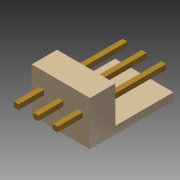
# Autodesk Inventor part: stiftleiste
Saved by Autodesk Inventor 2015 (Build 190159000, 159)
## iProperties
Created: 2015-03-02
Part Number: stiftleiste
Material: Generisch
Document SubType Name: Modeling
Designer: TowerSebi
Density: 1 g/cm^3
Appearance: Vorgabe
Author: TowerSebi
Autodesk Inventor part; units mm, degrees
ref_plane "YZ Plane" through (0, 0, 0) normal (1, 0, 0) x (0, 1, 0)
ref_plane "XZ Plane" through (0, 0, 0) normal (0, 1, 0) x (-1, 0, 0)
ref_plane "XY Plane" through (0, 0, 0) normal (0, 0, 1) x (1, 0, 0)
sketch "Skizze1" plane through (0, 0, 0) normal (0, 0, 1) x (1, 0, 0)
  line L0 (0, 0) -> (7.62, 0)
  line L1 (7.62, 0) -> (7.62, 3.3)
  line L2 (7.62, 3.3) -> (0, 3.3)
  line L3 (0, 3.3) -> (0, 0)
  dimension "d0" = 7.62
  dimension "d1" = 3.3
  constraints: 8 end point, 2 parallel, 1 horizontal, 1 perpendicular
  measures "d0" distance of L1.end L2.end
  measures "d1" distance of L2.end L0.start
extrude "Extrusion1" add sketch "Skizze1" along normal blind 5.8
sketch "Skizze2" plane through (0, 3.3, 0) normal (0, 1, 0) x (1, 0, 0)
  line L0 (7.62, 0) -> (7.62, -5.8) projected
  line L1 (0, 0) -> (7.62, 0)
  line L2 (7.62, 0) -> (7.62, -1)
  line L3 (7.62, -1) -> (0, -1)
  line L4 (0, -1) -> (0, 0)
  dimension "d4" = 1
  constraints: 8 end point, 2 parallel, 1 horizontal, 1 perpendicular, 1 point on line
  measures "d4" distance between parallel lines of L1 L3
extrude "Extrusion2" add sketch "Skizze2" along normal blind 7.6
sketch "Skizze3" plane through (0, 3.3, 5.8) normal (0, 1, 0) x (1, 0, 0)
  line L0 (7.62, 4.8) -> (0, 4.8) projected
  line L1 (0, 4.8) -> (0, 0) projected
  line L2 (7.62, 0) -> (0, 0) projected
  line L3 (7.62, 4.8) -> (7.62, 0) projected
  line L4 (0.95, 2.72) -> (1.59, 2.72)
  line L5 (1.59, 2.72) -> (1.59, 2.08)
  line L6 (1.59, 2.08) -> (0.95, 2.08)
  line L7 (0.95, 2.08) -> (0.95, 2.72)
  line L8 (3.49, 2.72) -> (4.13, 2.72)
  line L9 (4.13, 2.72) -> (4.13, 2.08)
  line L10 (4.13, 2.08) -> (3.49, 2.08)
  line L11 (3.49, 2.08) -> (3.49, 2.72)
  line L12 (6.03, 2.72) -> (6.67, 2.72)
  line L13 (6.67, 2.72) -> (6.67, 2.08)
  line L14 (6.67, 2.08) -> (6.03, 2.08)
  line L15 (6.03, 2.08) -> (6.03, 2.72)
  point P0 (0, 5.8)
  dimension "d7" = 0.64
  dimension "d8" = 0.64
  dimension "d9" = 0.64
  dimension "d10" = 0.64
  dimension "d11" = 0.64
  dimension "d12" = 0.64
  dimension "d13" = 7.62
  dimension "d15" = 1.9
  dimension "d16" = 1.9
  dimension "d17" = 0.95
  dimension "d18" = 0.95
  dimension "d19" = 4.8
  dimension "d20" = 2.08
  constraints: 24 end point, 6 parallel, 3 horizontal, 3 perpendicular
  measures "d7" distance of L14.end L12.start
  measures "d8" distance between parallel lines of L10 L8
  measures "d9" distance between parallel lines of L6 L4
  measures "d10" distance of L5.end L6.end
  measures "d11" distance of L13.end L14.end
  measures "d12" distance of L9.end L10.end
  measures "d13" distance between parallel lines of L3 L1
  measures "d15" distance between parallel lines of L11 L5
  measures "d16" distance between parallel lines of L15 L9
  measures "d17" distance between parallel lines of L1 L7
  measures "d18" distance between parallel lines of L3 L13
  measures "d19" distance between parallel lines of L2 L0
  measures "d20" distance between parallel lines of L6 L2
extrude "Extrusion3" add sketch "Skizze3" along normal blind 7.6 contours L4 L5 L6 L7 | L8 L9 L10 L11 | L12 L13 L14 L15
sketch "Skizze4" plane through (0, 0, 0) normal (0, -1, 0) x (1, 0, 0)
  line L0 (7.62, 0) -> (7.62, 5.8) projected
  line L1 (0, 5.8) -> (7.62, 5.8) projected
  line L2 (0, 0) -> (0, 5.8) projected
  line L3 (0.95, 3.72) -> (1.59, 3.72)
  line L4 (1.59, 3.72) -> (1.59, 3.08)
  line L5 (1.59, 3.08) -> (0.95, 3.08)
  line L6 (0.95, 3.08) -> (0.95, 3.72)
  line L7 (3.49, 3.72) -> (4.13, 3.72)
  line L8 (4.13, 3.72) -> (4.13, 3.08)
  line L9 (4.13, 3.08) -> (3.49, 3.08)
  line L10 (3.49, 3.08) -> (3.49, 3.72)
  line L11 (6.03, 3.72) -> (6.67, 3.72)
  line L12 (6.67, 3.72) -> (6.67, 3.08)
  line L13 (6.67, 3.08) -> (6.03, 3.08)
  line L14 (6.03, 3.08) -> (6.03, 3.72)
  dimension "d23" = 0.64
  dimension "d24" = 0.64
  dimension "d25" = 0.64
  dimension "d26" = 0.64
  dimension "d27" = 0.64
  dimension "d28" = 0.64
  dimension "d29" = 0.95
  dimension "d30" = 0.95
  dimension "d31" = 1.9
  dimension "d32" = 1.9
  dimension "d33" = 2.08
  dimension "d34" = 2.08
  dimension "d35" = 2.08
  constraints: 24 end point, 6 parallel, 3 horizontal, 3 perpendicular
  measures "d23" distance between parallel lines of L4 L6
  measures "d24" distance of L7.start L7.end
  measures "d25" distance of L11.start L11.end
  measures "d26" distance of L11.end L12.end
  measures "d27" distance of L7.end L8.end
  measures "d28" distance of L3.end L4.end
  measures "d29" distance between parallel lines of L6 L2
  measures "d30" distance between parallel lines of L0 L12
  measures "d31" distance between parallel lines of L10 L4
  measures "d32" distance between parallel lines of L14 L8
  measures "d33" distance between parallel lines of L3 L1
  measures "d34" distance between parallel lines of L1 L7
  measures "d35" distance between parallel lines of L1 L11
extrude "Extrusion4" add sketch "Skizze4" along normal blind 3.3
